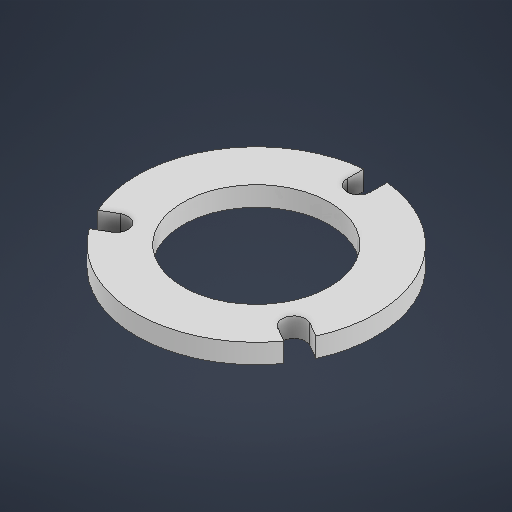
# Autodesk Inventor part: P_Lagerschale_Deckel
Saved by Autodesk Inventor 2026 (Build 300175000, 175)
## iProperties
Created: 2025-04-25
Part Number: P_Lagerschale_Deckel
Material: Generisch
Document SubType Name: Modeling
Designer: FAL
Density: 1 g/cm^3
Appearance: Vorgabe
Author: FAL
Autodesk Inventor part; units mm, degrees
ref_plane "YZ Plane" through (0, 0, 0) normal (1, 0, 0) x (0, 1, 0)
ref_plane "XZ Plane" through (0, 0, 0) normal (0, 1, 0) x (-1, 0, 0)
ref_plane "XY Plane" through (0, 0, 0) normal (0, 0, 1) x (1, 0, 0)
sketch "Skizze1" plane through (0, 0, 0) normal (0, 0, 1) x (1, 0, 0)
  circle A0 centre (0, 0) radius 12.25
  circle A1 centre (0, 0) radius 7.5
  dimension "d0" = 15
  dimension "d1" = 24.5
  constraints: 2 centre point, 2 coincident
  measures "d0" diameter of A1
  measures "d1" diameter of A0
extrude "Extrusion1" add sketch "Skizze1" along normal blind 2
sketch "Skizze2" plane through (0, 0, 2) normal (0, 0, 1) x (1, 0, 0)
  circle A0 centre (0, 0) radius 12.25 projected
  circle A1 centre (0, 0) radius 7.5 projected
  arc A2 (-1.2, 10.5) -> (1.2, 10.5) centre (0, 10.5) ccw
  line L0 (-1.2, 10.5) -> (-1.2, 13.3719)
  line L1 (-1.2, 13.3719) -> (1.2, 13.3719)
  line L2 (1.2, 13.3719) -> (1.2, 10.5)
  line L3 (0, 12.25) -> (0, 7.5)
  line L4 (0, -17.38) -> (0, 18.5303) projected
  dimension "d4" = 2.4
  dimension "d10" = 10.5
  constraints: 8 end point, 2 point on circle, 2 tangent, 2 vertical, 2 vertical alignment, 1 centre point, 1 collinear, 1 parallel, 1 perpendicular, 1 point on line, 2 other
  measures "d4" diameter of A2
  measures "d10" distance of point (0, 0) A2.centre
extrude "Extrusion2" cut sketch "Skizze2" against normal blind 2.4 contours L2 A2 L3 A0 | A0 L4 L1 L2 | L3 A2 L0 A0 | A0 L0 L1 L4
pattern_circular "Runde Anordnung1" count 3 over 360 about axis through (0, 0, 0) along (0, 0, 1) of "Extrusion2"
equation "\"d5\" = d4"
